Autodesk Fusion 360 part; units mm, degrees
note: some values were not read from the file. Set by a fixed rule: which face or edge a step refers to.
(part 3 of 4)
sketch "Sketch73" plane through (0, 0, 76.2) normal (0, 0, 1) x (1, 0, 0)
  line L0 (-231.5, 328) -> (-231.5, 317.5)
  line L1 (-231.5, 317.5) -> (-83.5, 317.5)
  line L2 (-83.5, 317.5) -> (-83.5, 328)
  line L3 (-83.5, 328) -> (-231.5, 328)
  circle A0 through (-77.5, 207.5, -7.5) (-80.5, 209.2321, -7.5) (-80.5, 205.7679, -7.5)
  circle A1 through (-77.5, 207.5, -7.5) (-80.5, 209.2321, -7.5) (-80.5, 205.7679, -7.5)
  circle A2 through (-77.5, 323.5, -7.5) (-80.5, 325.2321, -7.5) (-80.5, 321.7679, -7.5)
  circle A3 through (-77.5, 323.5, -7.5) (-80.5, 325.2321, -7.5) (-80.5, 321.7679, -7.5)
  circle A4 through (-233.5, 207.5, -25) (-236.5, 209.2321, -25) (-236.5, 205.7679, -25)
  circle A5 through (-233.5, 207.5, -25) (-236.5, 209.2321, -25) (-236.5, 205.7679, -25)
  circle A6 through (-233.5, 323.5, -25) (-236.5, 325.2321, -25) (-236.5, 321.7679, -25)
  circle A7 through (-233.5, 323.5, -25) (-236.5, 325.2321, -25) (-236.5, 321.7679, -25)
  circle A8 through (-77.5, 323.5, -25) (-80.5, 325.2321, -25) (-80.5, 321.7679, -25)
  circle A9 through (-77.5, 323.5, -25) (-80.5, 325.2321, -25) (-80.5, 321.7679, -25)
  circle A10 through (-77.5, 207.5, -25) (-80.5, 209.2321, -25) (-80.5, 205.7679, -25)
  circle A11 through (-77.5, 207.5, -25) (-80.5, 209.2321, -25) (-80.5, 205.7679, -25)
  point P0 (-235.5, 205.5)
sketch "Sketch74" plane through (0, 0, 76.2) normal (0, 0, 1) x (1, 0, 0)
  line L0 (-231.5, 213.5) -> (-231.5, 203)
  line L1 (-231.5, 203) -> (-83.5, 203)
  line L2 (-83.5, 203) -> (-83.5, 213.5)
  line L3 (-83.5, 213.5) -> (-231.5, 213.5)
  line L4 (-70, 213.5) -> (-140, 213.5)
  line L5 (-140, 213.5) -> (-140, 209.5)
  line L6 (-140, 209.5) -> (-70, 209.5)
  line L7 (-70, 209.5) -> (-70, 213.5)
  line L8 (-140, 209.5) -> (-175, 209.5)
  line L9 (-175, 209.5) -> (-175, 213.5)
  line L10 (-175, 213.5) -> (-140, 213.5)
  line L11 (-140, 213.5) -> (-140, 209.5)
  point P0 (-70, 213.5)
  dimension "d493" = 70
  dimension "d494" = 4
  dimension "d495" = 35
  constraint horizontal L4
  constraint vertical L5
  constraint horizontal L6
  constraint vertical L7
  constraint coincident P0 L4.start
  constraint horizontal L8
  constraint vertical L9
  constraint horizontal L10
  constraint vertical L11
  measures "d493" distance of P0 L4.end
  measures "d494" distance of P0 L6.end
  measures "d495" distance of L5.end L8.end
extrude "Extrude189" cut sketch "Sketch74" against normal blind 7.5 contours L3 L5 L8 L9 L10 L11 bodies 1
extrude "Extrude190" cut 1 faces at (-249.7333, 234.8333, 69.7) along direction (0, 0, 1) blind 2 on bodies 1 bodies 1
sketch "Sketch75" plane through (0, 213.5, 0) normal (0, 1, 0) x (-1, 0, 0)
  line L0 (175, 76.2) -> (175, 68.7)
  line L1 (175, 68.7) -> (140, 68.7)
  line L2 (140, 68.7) -> (140, 76.2)
  line L3 (140, 76.2) -> (83.5, 76.2)
  line L4 (83.5, 76.2) -> (83.5, 68.7)
  line L5 (83.5, 68.7) -> (74.5, 68.7)
  line L6 (74.5, 68.7) -> (74.5, 76.2)
  line L7 (74.5, 76.2) -> (70, 76.2)
  line L8 (70, 76.2) -> (70, 51.2)
  line L9 (245, 51.2) -> (245, 59.7)
  line L10 (245, 59.7) -> (267.2, 59.7)
  line L11 (267.2, 59.7) -> (257.6, 71.7)
  line L12 (257.6, 71.7) -> (245, 71.7)
  line L13 (245, 71.7) -> (245, 76.2)
  line L14 (245, 76.2) -> (240.5, 76.2)
  line L15 (240.5, 76.2) -> (240.5, 68.7)
  line L16 (240.5, 68.7) -> (231.5, 68.7)
  line L17 (231.5, 68.7) -> (231.5, 76.2)
  line L18 (231.5, 76.2) -> (175, 76.2)
extrude "Extrude191" cut 1 faces at (-252.4, 256.1667, 59.7) along direction (0, 0, -1) blind 2 on bodies 1 bodies 1
sketch "Sketch76" plane through (-192.0488, 0, 153.639) normal (-0.780869, 0, 0.624695) x (0.624695, 0, 0.780869)
  line L0 (-99.1703, 328) -> (-124.7828, 328)
  line L1 (-124.7828, 0) -> (-99.1703, 0)
  line L2 (-99.1703, 0) -> (-99.1703, 5)
  line L3 (-99.1703, 5) -> (-99.1703, 203)
  line L4 (-99.1703, 203) -> (-99.1703, 328)
  line L5 (-120.3006, 277.5) -> (-104.9332, 277.5)
  line L6 (-104.9332, 277.5) -> (-104.9332, 213.5)
  line L7 (-104.9332, 213.5) -> (-120.3006, 213.5)
sketch "Sketch77" plane through (0, 0, 57.7) normal (0, 0, 1) x (1, 0, 0)
  line L0 (-267.2, 277.5) -> (-267.2, 213.5)
  line L1 (-267.2, 213.5) -> (-245, 213.5)
  line L2 (-245, 213.5) -> (-245, 277.5)
  line L3 (-245, 277.5) -> (-267.2, 277.5)
  line L4 (-245, 213.5) -> (-254, 213.5)
  line L5 (-254, 213.5) -> (-254, 277.5)
  line L6 (-254, 277.5) -> (-245, 277.5)
  line L7 (-245, 277.5) -> (-245, 213.5)
  line L8 (-257.6, 213.5, 14) -> (-307.6, 213.5, 14)
  line L9 (-307.6, 213.5, 14) -> (-307.6, 277.5, 14)
  line L10 (-307.6, 277.5, 14) -> (-257.6, 277.5, 14)
  line L11 (-257.6, 277.5, 14) -> (-257.6, 213.5, 14)
  line L12 (-257.6, 277.5, 14) -> (-307.6, 277.5, 14)
  line L13 (-307.6, 277.5, 14) -> (-307.6, 287.5, 14)
  line L14 (-307.6, 287.5, 14) -> (-257.6, 287.5, 14)
  line L15 (-257.6, 287.5, 14) -> (-257.6, 277.5, 14)
  line L16 (-307.6, 213.5, 14) -> (-257.6, 213.5, 14)
  line L17 (-257.6, 213.5, 14) -> (-257.6, 203.5, 14)
  line L18 (-257.6, 203.5, 14) -> (-307.6, 203.5, 14)
  line L19 (-307.6, 203.5, 14) -> (-307.6, 213.5, 14)
  line L20 (-307.6, 287.5, 14) -> (-317.6, 287.5, 14)
  line L21 (-317.6, 287.5, 14) -> (-317.6, 203.5, 14)
  line L22 (-317.6, 203.5, 14) -> (-307.6, 203.5, 14)
  line L23 (-307.6, 203.5, 14) -> (-307.6, 287.5, 14)
  point P0 (-257.6, 213.5)
  dimension "d502" = 9
  dimension "d503" = 50
  dimension "d504" = 10
  dimension "d505" = 10
  dimension "d506" = 10
  constraint horizontal L4
  constraint vertical L5
  constraint horizontal L6
  constraint vertical L7
  constraint coincident L1.end L2.start
  measures "d502" distance of L1.end L4.end
extrude "Extrude192" add sketch "Sketch77" against normal blind 72 separate body contours L9 L13 L19 L20 L21 L22 L23 in plane through (0, 0, 71.7) normal (0, 0, 1) makes body 4
extrude "Extrude193" cut 1 faces at (-267.2, 234.8333, 59.0333) along direction (-1, 0, 0) blind 7 on bodies 1 bodies 1
sketch "Sketch78" plane through (0, 0, 71.7) normal (0, 0, 1) x (1, 0, 0)
  line L0 (-307.6, 203.5) -> (-307.6, 287.5)
  line L1 (-307.6, 287.5) -> (-317.6, 287.5)
  line L2 (-317.6, 287.5) -> (-317.6, 203.5)
  line L3 (-317.6, 203.5) -> (-307.6, 203.5)
  line L4 (-257.6, 277.5) -> (-307.6, 277.5)
  line L5 (-257.6, 213.5) -> (-307.6, 213.5)
  line L6 (-257.6, 213.5, 0) -> (-268.8, 213.5, -14)
  line L7 (-307.6, 277.5) -> (-268.8, 277.5)
  line L8 (-268.8, 277.5, 0) -> (-268.8, 277.5, -14)
  line L9 (-268.8, 277.5, -14) -> (-307.6, 277.5, -14)
  line L10 (-307.6, 277.5, -14) -> (-307.6, 277.5, 0)
  line L11 (-307.6, 213.5) -> (-268.8, 213.5)
  line L12 (-268.8, 213.5, 0) -> (-268.8, 213.5, -14)
  line L13 (-268.8, 213.5, -14) -> (-307.6, 213.5, -14)
  line L14 (-307.6, 213.5, -14) -> (-307.6, 213.5, 0)
  point P0 (-257.6, 277.5)
  point P1 (-257.6, 213.5)
  point P2 (-257.6, 213.5)
  point P3 (-268.8, 213.5)
  point P4 (-268.8, 277.5)
  constraint coincident P0 L4.start
  constraint coincident L0 L4.end
  constraint perpendicular L0 L4
  constraint coincident P2 P1
  constraint coincident L0 L5.end
  constraint perpendicular L0 L5
  constraint coincident P3 L11.end
  constraint horizontal L7
  constraint coincident P4 L7.end
  constraint horizontal L11
extrude "Extrude194" add sketch "Sketch78" against normal blind 10 contours L5 L6 L12 | L5 L11 L12 L13 L14 in plane through (0, 213.5, 71.7) normal (0, 1, 0) bodies 4 1
sketch "Sketch79" plane through (0, 287.5, 0) normal (0, 1, 0) x (-1, 0, 0)
  line L0 (317.6, 71.7) -> (307.6, 71.7)
  line L1 (307.6, 71.7) -> (307.6, -0.3)
  line L2 (307.6, -0.3) -> (317.6, -0.3)
  line L3 (317.6, -0.3) -> (317.6, 71.7)
  line L4 (307.6, 71.7, -74) -> (307.6, 71.7, 0)
  line L5 (257.6, 71.7, -10) -> (307.6, 71.7, -10)
  line L6 (268.8, 57.7, -10) -> (257.6, 71.7, -10)
  line L7 (268.8, 57.7, -10) -> (307.6, 57.7, -10)
  line L8 (307.6, 57.7, -10) -> (307.6, 71.7, -10)
  line L9 (307.6, 71.7, -10) -> (268.8, 71.7, -10)
  line L10 (268.8, 71.7, -10) -> (268.8, 57.7, -10)
  point P0 (257.6, 71.7)
  point P1 (268.8, 57.7)
  point P2 (257.6, 71.7)
  constraint coincident P2 P0
extrude "Extrude195" add sketch "Sketch79" along normal blind 10 separate body contours L5 L6 L10 | L5 L7 L8 L9 L10 in plane through (0, 277.5, 0) normal (0, 1, 0) makes body 5
sketch "Sketch80" plane through (-317.6, 0, 0) normal (-1, 0, 0) x (0, 0, 1)
sketch "Sketch81" plane through (0, 203.5, 0) normal (0, -1, 0) x (1, 0, 0)
  line L0 (-257.6, 71.7) -> (-317.6, 71.7)
  line L1 (-317.6, 71.7) -> (-317.6, -0.3)
  line L2 (-317.6, -0.3) -> (-307.6, -0.3)
  line L3 (-307.6, -0.3) -> (-307.6, 57.7)
  line L4 (-307.6, 57.7) -> (-268.8, 57.7)
  line L5 (-268.8, 57.7) -> (-257.6, 71.7)
  line L6 (-268.8, 57.7) -> (-307.6, 57.7)
  line L7 (-270, 56.2, -124.5) -> (-270, 56.2, 203.5)
  line L8 (-268.8, 57.7) -> (-270, 56.2)
  line L9 (-307.6, 57.7) -> (-270, 57.7)
  line L10 (-270, 57.7) -> (-270, 56.2)
  line L11 (-270, 56.2) -> (-307.6, 56.2)
  line L12 (-307.6, 56.2) -> (-307.6, 57.7)
  line L13 (-279, 0, -124.5) -> (-279, 10, -124.5)
  line L14 (-279, 10, -124.5) -> (-279, 10, -84)
  line L15 (-279, 10, -84) -> (-279, 0, -84)
  line L16 (-279, 0, -84) -> (-279, 0, -124.5)
  line L17 (-279, 0, -84) -> (-317.6, 0, -84)
  line L18 (-317.6, 0, -84) -> (-317.6, 10, -84)
  line L19 (-317.6, 10, -84) -> (-279, 10, -84)
  line L20 (-279, 10, -84) -> (-279, 0, -84)
  line L21 (-307.6, 10, -84) -> (-307.6, 0, -84)
  point P0 (-279, 0)
  dimension "d515" = 10
  dimension "d516" = 40.5
  dimension "d517" = 10
  constraint coincident L4.end L5.start
  constraint coincident L3.end L4.start
  constraint parallel L5 L8
  constraint horizontal L9
  constraint vertical L10
  constraint horizontal L11
  constraint vertical L12
extrude "Extrude196" add sketch "Sketch81" along normal blind 84.001 separate body contours L15 L17 L19 L20 L21 in plane through (0, 287.5, 0) normal (0, -1, 0) makes body 6
sketch "Sketch82" plane through (0, 0, 76.2) normal (0, 0, 1) x (1, 0, 0)
  line L0 (-240.5, 203) -> (-240.5, 213.5)
  line L1 (-240.5, 213.5) -> (-245, 213.5)
  line L2 (-245, 213.5) -> (-245, 317.5)
  line L3 (-245, 317.5) -> (-240.5, 317.5)
  line L4 (-240.5, 317.5) -> (-240.5, 328)
  line L5 (-240.5, 328) -> (-254, 328)
  line L6 (-254, 328) -> (-254, 203)
  line L7 (-254, 203) -> (-240.5, 203)
  line L8 (-245, 277.5, -18.5) -> (-307.6, 277.5, -18.5)
  line L9 (-307.6, 277.5, -18.5) -> (-307.6, 213.5, -18.5)
  line L10 (-307.6, 213.5, -18.5) -> (-245, 213.5, -18.5)
  line L11 (-245, 213.5, -18.5) -> (-245, 277.5, -18.5)
  point P0 (-245, 277.5)
  point P1 (-307.6, 213.5)
extrude "Extrude197" cut sketch "Sketch82" against normal blind 50 contours L8 L9 L10 L11 in plane through (0, 0, 57.7) normal (0, 0, 1) bodies 4 6
sketch "Sketch83" plane through (0, 213.5, 0) normal (0, 1, 0) x (-1, 0, 0)
  line L0 (175, 76.2) -> (175, 68.7)
  line L1 (175, 68.7) -> (140, 68.7)
  line L2 (140, 68.7) -> (140, 76.2)
  line L3 (140, 76.2) -> (83.5, 76.2)
  line L4 (83.5, 76.2) -> (83.5, 68.7)
  line L5 (83.5, 68.7) -> (74.5, 68.7)
  line L6 (74.5, 68.7) -> (74.5, 76.2)
  line L7 (74.5, 76.2) -> (70, 76.2)
  line L8 (70, 76.2) -> (70, 51.2)
  line L9 (70, 51.2) -> (254, 51.2)
  line L10 (254, 51.2) -> (254, 20)
  line L11 (254, 20) -> (245, 20)
  line L12 (245, 20) -> (245, 15.5)
  line L13 (245, 15.5) -> (247, 15.5)
  line L14 (247, 15.5) -> (247, 10)
  line L15 (247, 10) -> (254, 10)
  line L16 (254, 10) -> (254, 7.7)
  line L17 (254, 7.7) -> (279, 7.7)
  line L18 (279, 7.7) -> (279, 36.1286)
  line L19 (279, 36.1286) -> (270, 45.1607)
  line L20 (270, 45.1607) -> (270, 56.2)
  line L21 (270, 56.2) -> (268.8, 57.7)
  line L22 (268.8, 57.7) -> (307.6, 57.7)
  line L23 (307.6, 57.7) -> (307.6, 71.7)
  line L24 (307.6, 71.7) -> (257.6, 71.7)
  line L25 (257.6, 71.7) -> (245, 71.7)
  line L26 (245, 71.7) -> (245, 76.2)
  line L27 (245, 76.2) -> (240.5, 76.2)
  line L28 (240.5, 76.2) -> (240.5, 68.7)
  line L29 (240.5, 68.7) -> (231.5, 68.7)
  line L30 (231.5, 68.7) -> (231.5, 76.2)
  line L31 (231.5, 76.2) -> (175, 76.2)
  line L32 (279, 10) -> (307.6, 10)
  line L33 (307.6, 10) -> (307.6, 57.7)
  line L34 (307.6, 57.7) -> (279, 57.7)
  line L35 (279, 57.7) -> (279, 10)
  point P0 (279, 10)
  constraint horizontal L32
  constraint vertical L33
  constraint horizontal L34
  constraint vertical L35
  constraint coincident L22.end L23.start
  constraint coincident P0 L32.start
extrude "Extrude198" add sketch "Sketch83" against normal blind 10 contours L18 L22 L32 L33 L34 L35 bodies 6 5 4
sketch "Sketch84" plane through (0, 213.5, 0) normal (0, 1, 0) x (-1, 0, 0)
  line L0 (307.6, 7.7) -> (307.6, 71.7)
  line L1 (307.6, 71.7) -> (257.6, 71.7)
  line L2 (257.6, 71.7) -> (245, 71.7)
  line L3 (245, 71.7) -> (245, 76.2)
  line L4 (245, 76.2) -> (240.5, 76.2)
  line L5 (240.5, 76.2) -> (240.5, 68.7)
  line L6 (240.5, 68.7) -> (231.5, 68.7)
  line L7 (231.5, 68.7) -> (231.5, 76.2)
  line L8 (231.5, 76.2) -> (175, 76.2)
  line L9 (175, 76.2) -> (175, 68.7)
  line L10 (175, 68.7) -> (140, 68.7)
  line L11 (140, 68.7) -> (140, 76.2)
  line L12 (140, 76.2) -> (83.5, 76.2)
  line L13 (83.5, 76.2) -> (83.5, 68.7)
  line L14 (83.5, 68.7) -> (74.5, 68.7)
  line L15 (74.5, 68.7) -> (74.5, 76.2)
  line L16 (74.5, 76.2) -> (70, 76.2)
  line L17 (70, 76.2) -> (70, 51.2)
  line L18 (70, 51.2) -> (254, 51.2)
  line L19 (254, 51.2) -> (254, 20)
  line L20 (254, 20) -> (245, 20)
  line L21 (245, 20) -> (245, 15.5)
  line L22 (245, 15.5) -> (247, 15.5)
  line L23 (247, 15.5) -> (247, 10)
  line L24 (247, 10) -> (254, 10)
  line L25 (254, 10) -> (254, 7.7)
  line L26 (254, 7.7) -> (307.6, 7.7)
  line L27 (279, 36.1286) -> (270, 45.1607)
  line L28 (270, 56.2) -> (268.8, 57.7)
  line L29 (268.8, 57.7) -> (279, 57.7)
extrude "Extrude199" cut 1 faces at (-275.6, 206.8333, 57.7) along direction (0, 0, -1) blind 2 on bodies 6 bodies 6
extrude "Extrude200" add 1 faces at (-275.6, 206.8333, 57.7) along direction (0, 0, -1) blind 2 on bodies 6 bodies 6
sketch "Sketch85" plane through (0, 203.5, 0) normal (0, -1, 0) x (1, 0, 0)
  line L0 (-257.6, 71.7) -> (-317.6, 71.7)
  line L1 (-317.6, 71.7) -> (-317.6, -0.3)
  line L2 (-317.6, -0.3) -> (-307.6, -0.3)
  line L3 (-307.6, -0.3) -> (-307.6, 0)
  line L4 (-307.6, 0) -> (-307.6, 10)
  line L5 (-307.6, 10) -> (-279, 10)
  line L6 (-279, 10) -> (-279, 36.1286)
  line L7 (-279, 36.1286) -> (-279, 55.7)
  line L8 (-279, 55.7) -> (-270, 55.7)
  line L9 (-270, 55.7) -> (-270, 56.2)
  line L10 (-270, 56.2) -> (-257.6, 71.7)
  line L11 (-270, 55.7) -> (-279, 55.7)
  line L12 (-279, 55.7) -> (-279, 36.1286)
  line L13 (-270, 45.1607, 203.5) -> (-270, 45.1607, -10)
  line L14 (-279, 36.1286) -> (-270, 45.1607)
  line L15 (-270, 55.7) -> (-270, 45.1607)
  constraint coincident L8.end L9.start
  constraint coincident L7.end L8.start
  constraint coincident L6.end L7.start
extrude "Extrude201" add sketch "Sketch85" against normal blind 10 separate body contours L7 L8 L11 L12 L14 L15 makes body 7
extrude "Extrude202" cut 3 faces at (-301.4, 203.5, 39.2762) (-288.5333, 203.4993, 10) (-307.6, 203.4997, 6.6667) along direction (0, 1, 0) blind 3 on bodies 6 bodies 6
extrude "Extrude203" cut 1 faces at (-298.0667, 203.499, 6.6667) along direction (0, 1, 0) blind 3 on bodies 6 bodies 6
extrude "Extrude204" cut 1 faces at (-276, 203.5, 45.6631) along direction (0, 1, 0) blind 3 on bodies 7 bodies 7
extrude "Extrude205" cut 1 faces at (-317.6, 260.5, 23.7) along direction (1, 0, 0) blind 3 on bodies 6 bodies 6
sketch "Sketch86" plane through (0, 213.5, 0) normal (0, 1, 0) x (-1, 0, 0)
  line L0 (279, 10, 74) -> (307.6, 10, 74)
  line L1 (307.6, 10, 74) -> (307.6, 57.7, 74)
  line L2 (307.6, 57.7, 74) -> (279, 57.7, 74)
  line L3 (279, 57.7, 74) -> (279, 10, 74)
  line L4 (268.8, 57.7, 74) -> (279, 57.7, 74)
  point P0 (279, 10)
  point P1 (307.6, 57.7)
  point P2 (268.8, 57.7)
extrude "Extrude206" add sketch "Sketch86" against normal blind 10 contours L0 L1 L2 L3 in plane through (0, 287.5, 0) normal (0, 1, 0) bodies 5 7 6
sketch "Sketch87" plane through (0, 287.5, 0) normal (0, 1, 0) x (-1, 0, 0)
  line L0 (268.8, 57.7) -> (279, 57.7)
  line L1 (279, 57.7) -> (279, 36.1286)
  line L2 (279, 36.1286) -> (279, 0)
  line L3 (279, 0) -> (307.6, 0)
  line L4 (307.6, 0) -> (307.6, -0.3)
  line L5 (307.6, -0.3) -> (314.6, -0.3)
  line L6 (314.6, -0.3) -> (314.6, 71.7)
  line L7 (314.6, 71.7) -> (257.6, 71.7)
  line L8 (257.6, 71.7) -> (268.8, 57.7)
  line L9 (268.8, 57.7, -10) -> (268.8, 57.7, 0)
  line L10 (268.8, 57.7) -> (270, 56.2)
  line L11 (270, 56.2) -> (270, 57.7)
  point P0 (270, 45.1607)
  point P1 (270, 45.1607)
  point P2 (270, 56.2)
  point P3 (270, 56.2)
  point P4 (268.8, 57.7)
  constraint coincident P4 L0.start
  constraint parallel L8 L10
  constraint coincident L0 L11.end
  constraint perpendicular L0 L11
extrude "Extrude207" add sketch "Sketch87" against normal blind 10 separate body contours L0 L10 L11 makes body 8
sketch "Sketch88" plane through (0, 287.5, 0) normal (0, 1, 0) x (-1, 0, 0)
  line L0 (279, 36.1286) -> (279, 0)
  line L1 (279, 0) -> (307.6, 0)
  line L2 (307.6, 0) -> (307.6, -0.3)
  line L3 (307.6, -0.3) -> (314.6, -0.3)
  line L4 (314.6, -0.3) -> (314.6, 71.7)
extrude "Extrude208" add 1 faces at (-270, 284.1667, 56.7) along direction (-1, 0, 0) blind 9 on bodies 8 bodies 8 7 5
extrude "Extrude209" add 1 faces at (-270, 297.6667, 48.8405) along direction (-1, 0, 0) blind 9 on bodies 8 bodies 8
sketch "Sketch89" plane through (0, 328, 0) normal (0, 1, 0) x (-1, 0, 0)
  line L0 (231.5, 68.7) -> (231.5, 76.2)
  line L1 (231.5, 76.2) -> (83.5, 76.2)
  line L2 (83.5, 76.2) -> (83.5, 68.7)
  line L3 (83.5, 68.7) -> (74.5, 68.7)
  line L4 (74.5, 68.7) -> (74.5, 76.2)
  line L5 (74.5, 76.2) -> (61, 76.2)
  line L6 (61, 76.2) -> (45, 56.1607)
  line L7 (45, 56.1607) -> (53.7273, 56.1821)
  line L8 (53.7273, 56.1821) -> (51, 56.1607)
  line L9 (51, 56.1607) -> (45, 56.1607)
  line L10 (45, 56.1607) -> (45, 45.1607)
  line L11 (45, 45.1607) -> (36, 36.1286)
  line L12 (36, 36.1286) -> (36, 0)
  line L13 (36, 0) -> (56, 0)
  line L14 (56, 0) -> (56, -71)
  line L15 (56, -71) -> (61, -71)
  line L16 (61, -71) -> (61, 51.2)
  line L17 (61, 51.2) -> (254, 51.2)
  line L18 (254, 51.2) -> (254, -71)
  line L19 (254, -71) -> (259, -71)
  line L20 (259, -71) -> (259, 0)
  line L21 (259, 0) -> (279, 0)
  line L22 (279, 0) -> (279, 36.1286)
  line L23 (279, 36.1286) -> (270, 45.1607)
  line L24 (270, 45.1607) -> (279, 45.1607)
  line L25 (279, 45.1607) -> (279, 56.2)
  line L26 (279, 56.2) -> (270, 56.2)
  line L27 (270, 56.2) -> (254, 76.2)
  line L28 (254, 76.2) -> (240.5, 76.2)
  line L29 (240.5, 76.2) -> (240.5, 68.7)
  line L30 (240.5, 68.7) -> (231.5, 68.7)
  line L31 (270, 56.2) -> (279, 56.2)
  line L32 (279, 56.2) -> (279, 36.1286)
  line L33 (279, 36.1286) -> (270, 36.1286)
  line L34 (270, 36.1286) -> (270, 56.2)
  line L35 (270, 45.1607) -> (279, 45.1607)
  line L36 (270, 45.1607) -> (279, 36.1286)
  constraint horizontal L31
  constraint vertical L32
  constraint horizontal L33
  constraint vertical L34
  constraint coincident L22.end L23.start
  constraint coincident L26.end L27.start
  constraint coincident L23.end L24.start
  constraint coincident L24.end L25.start
extrude "Extrude210" add sketch "Sketch89" against normal blind 50.5 separate body contours L23 L24 L32 L35 L36 makes body 9
sketch "Sketch90" plane through (0, 328, 0) normal (0, 1, 0) x (-1, 0, 0)
  line L0 (231.5, 68.7) -> (231.5, 76.2)
  line L1 (231.5, 76.2) -> (83.5, 76.2)
  line L2 (83.5, 76.2) -> (83.5, 68.7)
  line L3 (83.5, 68.7) -> (74.5, 68.7)
  line L4 (74.5, 68.7) -> (74.5, 76.2)
  line L5 (74.5, 76.2) -> (61, 76.2)
  line L6 (61, 76.2) -> (45, 56.1607)
  line L7 (45, 56.1607) -> (53.7273, 56.1821)
  line L8 (53.7273, 56.1821) -> (51, 56.1607)
  line L9 (51, 56.1607) -> (45, 56.1607)
  line L10 (45, 56.1607) -> (45, 45.1607)
  line L11 (45, 45.1607) -> (36, 36.1286)
  line L12 (36, 36.1286) -> (36, 0)
  line L13 (36, 0) -> (56, 0)
  line L14 (56, 0) -> (56, -71)
  line L15 (56, -71) -> (61, -71)
  line L16 (61, -71) -> (61, 51.2)
  line L17 (61, 51.2) -> (254, 51.2)
  line L18 (254, 51.2) -> (254, -71)
  line L19 (254, -71) -> (259, -71)
  line L20 (259, -71) -> (259, 0)
  line L21 (259, 0) -> (279, 0)
  line L22 (279, 0) -> (279, 36.1286)
  line L23 (279, 36.1286) -> (270, 45.1607)
  line L24 (270, 45.1607) -> (279, 45.1607)
  line L25 (279, 45.1607) -> (279, 56.2)
  line L26 (279, 56.2) -> (270, 56.2)
  line L27 (270, 56.2) -> (254, 76.2)
  line L28 (254, 76.2) -> (240.5, 76.2)
  line L29 (240.5, 76.2) -> (240.5, 68.7)
  line L30 (240.5, 68.7) -> (231.5, 68.7)
  line L31 (279, 56.2) -> (259, 56.2)
  line L32 (259, 56.2) -> (259, 0)
  line L33 (259, 0) -> (279, 0)
  line L34 (279, 0) -> (279, 56.2)
  constraint horizontal L31
  constraint vertical L32
  constraint horizontal L33
  constraint vertical L34
  constraint coincident L20.end L21.start
  constraint coincident L25.end L26.start
extrude "Extrude211" cut sketch "Sketch90" against normal blind 40 contours L21 L22 L23 L24 L25 L26 L31 L32 L33 L34 | L23 L24 L34 bodies 8 9
extrude "Extrude212" cut 1 faces at (-272.3333, 288, 12.0429) along direction (0, -1, 0) blind 10 on bodies 8 bodies 8
extrude "Extrude213" cut 1 faces at (-276, 288, 42.15) along direction (0, -1, 0) blind 10 on bodies 9 bodies 9
extrude "Extrude214" cut 1 faces at (-272.3333, 278, 12.0429) along direction (0, -1, 0) blind 3 on bodies 8 bodies 8
extrude "Extrude215" cut 1 faces at (-276, 277.5, 42.15) along direction (0, 1, 0) blind 2 on bodies 9 bodies 9
extrude "Extrude216" cut 1 faces at (-262.6667, 297.6667, 56.2) along direction (0, 0, 1) blind 20 on bodies 8 bodies 8
extrude "Extrude217" add 1 faces at (-265.6667, 275, 5.1333) along direction (0, 1, 0) blind 12.5 on bodies 8 bodies 8 9
sketch "Sketch91" plane through (0, 287.5, 0) normal (0, 1, 0) x (-1, 0, 0)
  line L0 (259, 69.95) -> (259, 71.7)
  line L1 (259, 69.95) -> (257.6, 71.7)
  line L2 (257.6, 71.7) -> (259, 71.7)
  point P0 (259, 69.95)
  point P1 (259, 71.7)
  point P2 (257.6, 71.7)
  constraint coincident P0 L0.start
  constraint coincident P1 L0.end
  constraint coincident P2 L1.end
extrude "Extrude218" cut sketch "Sketch91" against normal blind 11.8 bodies 8
extrude "Extrude219" add 1 faces at (-279, 284.1667, 50.3667) along direction (1, 0, 0) blind 20 on bodies 8 bodies 8
extrude "Extrude220" cut 1 faces at (-293.7333, 284.1667, 71.7) along direction (0, 0, -1) blind 2 on bodies 8 bodies 8
sketch "Sketch92" plane through (0, 0, 69.7) normal (0, 0, 1) x (1, 0, 0)
  line L0 (-259, 287.5) -> (-314.6, 287.5)
  line L1 (-314.6, 287.5) -> (-314.6, 206.5)
  line L2 (-314.6, 206.5) -> (-259.2, 206.5)
  line L3 (-259.2, 206.5) -> (-257.6, 206.5)
  line L4 (-257.6, 206.5) -> (-257.6, 213.5)
  line L5 (-257.6, 213.5) -> (-307.6, 213.5)
  line L6 (-307.6, 213.5) -> (-307.6, 277.5)
  line L7 (-307.6, 277.5) -> (-259, 277.5)
  line L8 (-259, 277.5) -> (-259, 287.5)
  line L9 (-257.6, 213.5) -> (-307.6, 213.5)
  line L10 (-307.6, 213.5) -> (-307.6, 277.5)
  line L11 (-307.6, 277.5) -> (-257.6, 277.5)
  line L12 (-257.6, 277.5) -> (-257.6, 213.5)
  constraint horizontal L9
  constraint vertical L10
  constraint horizontal L11
  constraint vertical L12
  constraint coincident L6.end L7.start
  constraint coincident L4.end L5.start
extrude "Extrude221" add sketch "Sketch92" along normal blind 5 separate body contours L5 L6 L7 L9 L10 L11 L12 makes body 10
extrude "Extrude222" cut 1 faces at (-274.7333, 234.8333, 74.7) along direction (0, 0, -1) blind 3 on bodies 10 bodies 10
extrude "Extrude223" add 1 faces at (-293.7333, 284.1667, 69.7) along direction (0, 0, 1) blind 2 on bodies 8 bodies 8 10
extrude "Extrude224" add 1 faces at (-258.5333, 277.5, 71.1167) along direction (0, 1, 0) blind 10 on bodies 8 bodies 8
extrude "Extrude225" cut 1 faces at (-281.8667, 260.4997, 0) along direction (0, 0, 1) blind 3 on bodies 8 bodies 8
extrude "Extrude226" cut 1 faces at (-312.2667, 260.5, -0.3) along direction (0, 0, 1) blind 3.3 on bodies 8 bodies 8
fillet "Fillet1" radius 8 1 edges at (-314.6, 247, 71.7) on bodies 8
fillet "Fillet2" radius 8 1 edges at (-314.6, 247, 3) on bodies 8
fillet "Fillet3" radius 8 5 edges at (-282.8, 287.5, 3) (-312.2569, 287.5, 5.3431) (-314.6, 287.5, 37.35) (-312.2569, 287.5, 69.3569) (-282.1, 287.5, 71.7) on bodies 8
fillet "Fillet4" radius 4 4 edges at (-282.1, 206.5, 71.7) (-312.2569, 206.5, 69.3569) (-314.6, 206.5, 37.35) (-312.6, 206.5, 5.7085) on bodies 8
sketch "Sketch93" plane through (0, 0, 51.2) normal (0, 0, -1) x (-1, 0, 0)
  line L0 (254, 213.5) -> (70, 213.5)
  line L1 (70, 213.5) -> (70, 317.5)
  line L2 (70, 317.5) -> (245, 317.5)
  line L3 (245, 317.5) -> (245, 277.5)
  line L4 (245, 277.5) -> (254, 277.5)
  line L5 (254, 277.5) -> (254, 328)
  line L6 (254, 328) -> (61, 328)
  line L7 (61, 328) -> (61, 155)
  line L8 (61, 155) -> (66, 155)
  line L9 (66, 155) -> (66, 5)
  line L10 (66, 5) -> (89, 5)
  line L11 (89, 5) -> (89, 155)
  line L12 (89, 155) -> (96, 155)
  line L13 (96, 155) -> (96, 64.5)
  line L14 (96, 64.5) -> (219, 64.5)
  line L15 (219, 64.5) -> (219, 155)
  line L16 (219, 155) -> (226.5, 155)
  line L17 (226.5, 155) -> (226.5, 135)
  line L18 (226.5, 135) -> (223, 135)
  line L19 (223, 135) -> (223, 60.5)
  line L20 (223, 60.5) -> (218, 60.5)
  line L21 (218, 60.5) -> (218, 5)
  line L22 (218, 5) -> (250.5, 5)
  line L23 (250.5, 5) -> (250.5, 155)
  line L24 (250.5, 155) -> (254, 155)
  line L25 (254, 155) -> (254, 213.5)
  circle A0 centre (235.5, 323.5) radius 2
  circle A1 centre (79.5, 323.5) radius 2
  circle A2 centre (229, 25) radius 6.15
  circle A3 centre (235.5, 207.5) radius 2
  circle A4 centre (79.5, 207.5) radius 2
  line L26 (254, 317.5) -> (61, 317.5)
  line L27 (61, 317.5) -> (61, 328)
  line L28 (61, 328) -> (254, 328)
  line L29 (254, 328) -> (254, 317.5)
  constraint horizontal L26
  constraint vertical L27
  constraint horizontal L28
  constraint vertical L29
  constraint coincident L6.end L7.start
  constraint coincident L5 L26.start
extrude "Extrude227" cut sketch "Sketch93" against normal blind 5 contours L2 L5 L6 L7 L26 L27 L28 L29 bodies 8
sketch "Sketch94" plane through (0, 0, 51.2) normal (0, 0, -1) x (-1, 0, 0)
  circle A0 centre (79.5, 207.5) radius 2
  circle A1 centre (235.5, 207.5) radius 2
  circle A2 centre (229, 25) radius 6.15
  line L0 (70, 317.5) -> (61, 317.5)
  line L1 (61, 317.5) -> (61, 155)
  line L2 (61, 155) -> (66, 155)
  line L3 (66, 155) -> (66, 5)
  line L4 (66, 5) -> (89, 5)
  line L5 (89, 5) -> (89, 155)
  line L6 (89, 155) -> (96, 155)
  line L7 (96, 155) -> (96, 64.5)
  line L8 (96, 64.5) -> (219, 64.5)
  line L9 (219, 64.5) -> (219, 155)
  line L10 (219, 155) -> (226.5, 155)
  line L11 (226.5, 155) -> (226.5, 135)
  line L12 (226.5, 135) -> (223, 135)
  line L13 (223, 135) -> (223, 60.5)
  line L14 (223, 60.5) -> (218, 60.5)
  line L15 (218, 60.5) -> (218, 5)
  line L16 (218, 5) -> (250.5, 5)
  line L17 (250.5, 5) -> (250.5, 155)
  line L18 (250.5, 155) -> (254, 155)
  line L19 (254, 155) -> (254, 213.5)
  line L20 (254, 213.5) -> (70, 213.5)
  line L21 (70, 213.5) -> (70, 317.5)
  line L22 (254, 213.5) -> (61, 213.5)
  line L23 (61, 213.5) -> (61, 201.5)
  line L24 (61, 201.5) -> (254, 201.5)
  line L25 (254, 201.5) -> (254, 213.5)
  dimension "d590" = 12
  constraint horizontal L22
  constraint vertical L23
  constraint horizontal L24
  constraint vertical L25
  constraint coincident L19.end L20.start
  measures "d590" distance of L19.end L24.end
extrude "Extrude228" add 1 faces at (-132.8333, 203, 60.3667) along direction (0, -1, 0) blind 10 on bodies 8 bodies 8
extrude "Extrude229" cut sketch "Sketch94" against normal blind 5 contours L1 L19 L20 L22 L23 L24 L25 bodies 8
extrude "Extrude230" cut 1 faces at (-64, 282.8333, 51.2) along direction (0, 0, 1) blind 5 on bodies 8 bodies 8
extrude "Extrude231" cut 1 faces at (-248, 304.1667, 51.2) along direction (0, 0, 1) blind 5 on bodies 8 bodies 8
extrude "Extrude232" add 1 faces at (-249.2, 234.8333, 71.7) along direction (0, 0, -1) blind 2 on bodies 8 bodies 8
sketch "Sketch95" plane through (0, 213.5, 0) normal (0, 1, 0) x (-1, 0, 0)
extrude "Extrude233" cut 1 faces at (-237.6667, 217, 15.1667) along direction (0, -1, 0) blind 3.5 on bodies 8 bodies 8
extrude "Extrude234" cut 1 faces at (-62.6667, 155, 30.4) along direction (0, -1, 0) blind 150 on bodies 8 bodies 8
sketch "Sketch96" plane through (0, 328, 0) normal (0, 1, 0) x (-1, 0, 0)
  line L0 (61, -71) -> (61, 56.2)
  line L1 (61, 56.2) -> (254, 56.2)
  line L2 (254, 56.2) -> (254, -71)
  line L3 (254, -71) -> (259, -71)
  line L4 (259, -71) -> (259, 69.95)
  line L5 (259, 69.95) -> (254, 76.2)
  line L6 (254, 76.2) -> (240.5, 76.2)
  line L7 (240.5, 76.2) -> (240.5, 68.7)
  line L8 (240.5, 68.7) -> (231.5, 68.7)
  line L9 (231.5, 68.7) -> (231.5, 76.2)
  line L10 (231.5, 76.2) -> (83.5, 76.2)
  line L11 (83.5, 76.2) -> (83.5, 68.7)
  line L12 (83.5, 68.7) -> (74.5, 68.7)
  line L13 (74.5, 68.7) -> (74.5, 76.2)
  line L14 (74.5, 76.2) -> (61, 76.2)
  line L15 (61, 76.2) -> (45, 56.1607)
  line L16 (45, 56.1607) -> (53.7273, 56.1821)
  line L17 (53.7273, 56.1821) -> (51, 56.1607)
  line L18 (51, 56.1607) -> (45, 56.1607)
  line L19 (45, 56.1607) -> (45, 45.1607)
  line L20 (45, 45.1607) -> (36, 36.1286)
  line L21 (36, 36.1286) -> (36, 0)
  line L22 (36, 0) -> (56, 0)
  line L23 (56, 0) -> (56, -71)
  line L24 (56, -71) -> (61, -71)
  line L25 (61, 56.2) -> (254, 56.2)
  line L26 (254, 56.2) -> (254, 61.2)
  line L27 (254, 61.2) -> (61, 61.2)
  line L28 (61, 61.2) -> (61, 56.2)
  dimension "d605" = 5
  constraint horizontal L25
  constraint vertical L26
  constraint horizontal L27
  constraint vertical L28
  constraint coincident L0.end L1.start
  measures "d605" distance of L0.end L27.end
extrude "Extrude235" add sketch "Sketch96" along normal blind 5 separate body contours L0 L2 L3 L4 L5 L6 L7 L8 L9 L10 L11 L12 L13 L14 L15 L19 L20 L21 L22 L23 L24 L26 L27 L28 makes body 11
sketch "Sketch97" plane through (0, 333, 0) normal (0, 1, 0) x (-1, 0, 0)
  line L0 (254, 61.2) -> (254, -71)
  line L1 (254, -71) -> (259, -71)
  line L2 (259, -71) -> (259, 69.95)
  line L3 (259, 69.95) -> (254, 76.2)
  line L4 (254, 76.2) -> (240.5, 76.2)
  line L5 (240.5, 76.2) -> (240.5, 68.7)
  line L6 (240.5, 68.7) -> (231.5, 68.7)
  line L7 (231.5, 68.7) -> (231.5, 76.2)
  line L8 (231.5, 76.2) -> (83.5, 76.2)
  line L9 (83.5, 76.2) -> (83.5, 68.7)
  line L10 (83.5, 68.7) -> (74.5, 68.7)
  line L11 (74.5, 68.7) -> (74.5, 76.2)
  line L12 (74.5, 76.2) -> (61, 76.2)
  line L13 (61, 76.2) -> (45, 56.1607)
  line L14 (45, 56.1607) -> (53.7273, 56.1821)
  line L15 (53.7273, 56.1821) -> (51, 56.1607)
  line L16 (51, 56.1607) -> (45, 56.1607)
  line L17 (45, 56.1607) -> (45, 45.1607)
  line L18 (45, 45.1607) -> (36, 36.1286)
  line L19 (36, 36.1286) -> (36, 0)
  line L20 (36, 0) -> (56, 0)
  line L21 (56, 0) -> (56, -71)
  line L22 (56, -71) -> (61, -71)
  line L23 (61, -71) -> (61, 61.2)
  line L24 (61, 61.2) -> (254, 61.2)
  line L25 (61, 61.2) -> (56, 61.2)
  line L26 (56, 61.2) -> (56, -71)
  line L27 (56, -71) -> (61, -71)
  line L28 (61, -71) -> (61, 61.2)
  constraint horizontal L25
  constraint vertical L26
  constraint horizontal L27
  constraint vertical L28
  constraint coincident L21.end L22.start
  constraint coincident L23.end L24.start
extrude "Extrude236" cut sketch "Sketch97" against normal blind 5 contours L21 L22 L23 L25 L26 L27 L28 bodies 11
sketch "Sketch98" plane through (0, 0, 76.2) normal (0, 0, 1) x (1, 0, 0)
  line L0 (-254, 333, -15) -> (-259, 333, -15)
  line L1 (-259, 333, -15) -> (-259, 333, -147.2)
  line L2 (-259, 333, -147.2) -> (-254, 333, -147.2)
  line L3 (-254, 333, -147.2) -> (-254, 333, -15)
  point P0 (-254, 333)
  point P1 (-259, 333)
extrude "Extrude237" cut sketch "Sketch98" against normal blind 5 contours L0 L1 L2 L3 in plane through (0, 333, 76.2) normal (0, 1, 0) bodies 11
sketch "Sketch99" plane through (-259, 0, 0) normal (-1, 0, 0) x (0, 0, 1)
  line L0 (11, 287.5) -> (63.7, 287.5)
  arc A0 (69.95, 284.4937) -> (63.7, 287.5) centre (63.7, 279.5) ccw
  line L1 (69.95, 284.4937) -> (69.95, 328)
  line L2 (69.95, 328) -> (-71, 328)
  line L3 (-71, 328) -> (-71, 0)
  line L4 (-71, 0) -> (3, 0)
  line L5 (3, 0) -> (3, 279.5)
  arc A1 (11, 287.5) -> (3, 279.5) centre (11, 279.5) ccw
  line L6 (61.2, 333) -> (-71, 333)
  line L7 (-71, 333) -> (-71, 328)
  line L8 (-71, 328) -> (61.2, 328)
  line L9 (61.2, 328) -> (61.2, 333)
  point P0 (61.2, 333)
  constraint horizontal L6
  constraint vertical L7
  constraint horizontal L8
  constraint vertical L9
  constraint coincident L2.end L3.start
  constraint coincident P0 L6.start
extrude "Extrude238" add sketch "Sketch99" along normal blind 5 separate body makes body 12
sketch "Sketch100" plane through (-245, 0, 0) normal (1, 0, 0) x (0, 0, -1)
  line L0 (-56.2, 277.5) -> (-56.2, 317.5)
  line L1 (-56.2, 317.5) -> (-76.2, 317.5)
  line L2 (-76.2, 317.5) -> (-76.2, 213.5)
  line L3 (-76.2, 213.5) -> (-69.7, 213.5)
  line L4 (-69.7, 213.5) -> (-69.7, 277.5)
  line L5 (-69.7, 277.5) -> (-56.2, 277.5)
  line L6 (-56.2, 317.5) -> (-69.7, 317.5)
  line L7 (-69.7, 317.5) -> (-69.7, 277.5)
  line L8 (-69.7, 277.5) -> (-56.2, 277.5)
  line L9 (-56.2, 277.5) -> (-56.2, 317.5)
  constraint horizontal L6
  constraint vertical L7
  constraint horizontal L8
  constraint vertical L9
  constraint coincident L4.end L5.start
  constraint coincident L0.end L1.start
extrude "Extrude239" cut sketch "Sketch100" against normal blind 5 contours L0 L1 L5 L6 L7 L8 L9 bodies 8
extrude "Extrude240" cut 1 faces at (-289.7333, 277.5, 44.5333) along direction (0, 1, 0) blind 5 on bodies 8 bodies 8
extrude "Extrude241" add 1 faces at (-64, 247.6667, 56.2) along direction (0, 0, -1) blind 5 on bodies 8 bodies 8
extrude "Extrude242" cut 1 faces at (-235.8832, 318.8352, 68.7) along direction (0, 0, -1) blind 5 on bodies 8 bodies 8
extrude "Extrude243" cut 1 faces at (-237.5, 329.6667, 68.7) along direction (0, 0, -1) blind 5 on bodies 11 bodies 11
extrude "Extrude244" cut 1 faces at (-80.5, 329.6667, 68.7) along direction (0, 0, -1) blind 5 on bodies 11 bodies 11
extrude "Extrude245" cut 1 faces at (-79.1168, 318.8352, 68.7) along direction (0, 0, -1) blind 5 on bodies 8 bodies 8
extrude "Extrude246" cut 1 faces at (-235.8333, 197.1667, 68.7) along direction (0, 0, -1) blind 5 on bodies 8 bodies 8
extrude "Extrude247" cut 1 faces at (-79.1667, 197.1667, 68.7) along direction (0, 0, -1) blind 5 on bodies 8 bodies 8
extrude "Extrude248" add 1 faces at (-290.2667, 233.5, 71.7) along direction (0, 0, 1) blind 5 on bodies 8 bodies 8
extrude "Extrude249" cut 1 faces at (-151.6667, 210.8333, 68.7) along direction (0, 0, -1) blind 15 on bodies 8 bodies 8
extrude "Extrude250" cut sketch "Sketch84" against normal blind 3 bodies 7 8
extrude "Extrude251" cut 1 faces at (-289.7333, 282.5, 42.8667) along direction (0, 1, 0) blind 15 on bodies 8 bodies 8 12
extrude "Extrude252" cut 1 faces at (-307.6, 237.1458, 29.4667) along direction (-1, 0, 0) blind 10 on bodies 8 bodies 8
extrude "Extrude253" cut 1 faces at (-275.6292, 258.9292, 7.7) along direction (0, 0, -1) blind 5 on bodies 8 bodies 8 12
sketch "Sketch101" plane through (0, 0, 69.7) normal (0, 0, -1) x (-1, 0, 0)
  line L0 (245, 317.5) -> (245, 213.5)
  line L1 (245, 213.5) -> (311.8915, 213.5)
  line L2 (311.8915, 213.5) -> (311.8915, 279.5)
  arc A0 (311.8915, 279.5) -> (306.6, 284.7915) centre (306.6, 279.5) ccw
  line L3 (306.6, 284.7915) -> (259, 284.7915)
  line L4 (259, 284.7915) -> (259, 297.5)
  line L5 (259, 297.5) -> (250, 297.5)
  line L6 (250, 297.5) -> (250, 317.5)
  line L7 (250, 317.5) -> (245, 317.5)
  line L8 (259, 284.7915) -> (259, 213.5)
  constraint coincident L3.end L4.start
  constraint coincident L1 L8.end
  constraint perpendicular L1 L8
extrude "Extrude254" cut sketch "Sketch101" against normal blind 10 contours L1 L2 A0 L3 L8 bodies 8 12
sketch "Sketch102" plane through (0, 210.5, 0) normal (0, 1, 0) x (-1, 0, 0)
  arc A0 (314.6, 63.7) -> (306.6, 71.7) centre (306.6, 63.7) ccw
  line L0 (306.6, 71.7) -> (257.6, 71.7)
  line L1 (257.6, 71.7) -> (245, 71.7)
  line L2 (245, 71.7) -> (245, 76.2)
  line L3 (245, 76.2) -> (240.5, 76.2)
  line L4 (240.5, 76.2) -> (240.5, 63.7)
  line L5 (240.5, 63.7) -> (231.5, 63.7)
  line L6 (231.5, 63.7) -> (231.5, 76.2)
  line L7 (231.5, 76.2) -> (175, 76.2)
  line L8 (175, 76.2) -> (175, 53.7)
  line L9 (175, 53.7) -> (140, 53.7)
  line L10 (140, 53.7) -> (140, 76.2)
  line L11 (140, 76.2) -> (83.5, 76.2)
  line L12 (83.5, 76.2) -> (83.5, 63.7)
  line L13 (83.5, 63.7) -> (74.5, 63.7)
  line L14 (74.5, 63.7) -> (74.5, 76.2)
  line L15 (74.5, 76.2) -> (70, 76.2)
  line L16 (70, 76.2) -> (70, 51.2)
  line L17 (70, 51.2) -> (254, 51.2)
  line L18 (254, 51.2) -> (254, 20)
  line L19 (254, 20) -> (245, 20)
  line L20 (245, 20) -> (245, 15.5)
  line L21 (245, 15.5) -> (247, 15.5)
  line L22 (247, 15.5) -> (247, 10)
  line L23 (247, 10) -> (254, 10)
  line L24 (254, 10) -> (254, 2.7)
  line L25 (254, 2.7) -> (259, 2.7)
  line L26 (259, 2.7) -> (259, 3)
  line L27 (259, 3) -> (306.6, 3)
  arc A1 (306.6, 3) -> (307.6, 3.0627) centre (306.6, 11) ccw
  arc A2 (307.6, 3.0627) -> (314.6, 11) centre (306.6, 11) ccw
  line L28 (314.6, 11) -> (314.6, 63.7)
  line L29 (270, 55.7) -> (279, 55.7)
  line L30 (279, 55.7) -> (279, 36.1286)
  line L31 (279, 36.1286) -> (270, 45.1607)
  line L32 (270, 45.1607) -> (270, 55.7)
  line L33 (264, 2.7) -> (264, 71.7)
  point P0 (264, 2.7)
  constraint coincident P0 L33.start
  constraint coincident L0 L33.end
  constraint perpendicular L0 L33
extrude "Extrude255" cut sketch "Sketch102" against normal blind 5 contours A0 L0 L27 A1 A2 L28 L33 | L29 L30 L31 L32 bodies 7 8
extrude "Extrude256" add 1 faces at (-246.5, 198.8333, 76.2) along direction (0, 0, 1) blind 10 on bodies 8 bodies 8 12 7 11
extrude "Extrude257" add 1 faces at (-245, 329.6667, 76.2) along direction (0, 0, 1) blind 10 on bodies 8 bodies 8
extrude "Extrude258" cut 1 faces at (-251.3333, 241.5, 69.7) along direction (0, 0, 1) blind 10 on bodies 8 bodies 8
extrude "Extrude259" cut 1 faces at (-262.3333, 289.0277, 69.7) along direction (0, 0, 1) blind 2 on bodies 12 bodies 12
extrude "Extrude260" add 1 faces at (-260.6667, 328, 67.0333) along direction (0, 1, 0) blind 5 on bodies 12 bodies 12 8
sketch "Sketch103" plane through (0, 210.5, 0) normal (0, 1, 0) x (-1, 0, 0)
  line L0 (264, 2.7) -> (264, 71.7)
  line L1 (264, 71.7) -> (257.6, 71.7)
  line L2 (257.6, 71.7) -> (245, 71.7)
  line L3 (245, 71.7) -> (245, 86.2)
  line L4 (245, 86.2) -> (240.5, 86.2)
  line L5 (240.5, 86.2) -> (240.5, 63.7)
  line L6 (240.5, 63.7) -> (231.5, 63.7)
  line L7 (231.5, 63.7) -> (231.5, 76.2)
  line L8 (231.5, 76.2) -> (175, 76.2)
  line L9 (175, 76.2) -> (175, 53.7)
  line L10 (175, 53.7) -> (140, 53.7)
  line L11 (140, 53.7) -> (140, 76.2)
  line L12 (140, 76.2) -> (83.5, 76.2)
  line L13 (83.5, 76.2) -> (83.5, 63.7)
  line L14 (83.5, 63.7) -> (74.5, 63.7)
  line L15 (74.5, 63.7) -> (74.5, 76.2)
  line L16 (74.5, 76.2) -> (70, 76.2)
  line L17 (70, 76.2) -> (70, 51.2)
  line L18 (70, 51.2) -> (254, 51.2)
  line L19 (254, 51.2) -> (254, 20)
  line L20 (254, 20) -> (245, 20)
  line L21 (245, 20) -> (245, 15.5)
  line L22 (245, 15.5) -> (247, 15.5)
  line L23 (247, 15.5) -> (247, 10)
  line L24 (247, 10) -> (254, 10)
  line L25 (254, 10) -> (254, 2.7)
  line L26 (254, 2.7) -> (264, 2.7)
  line L27 (254, 2.7) -> (264, 2.7)
  line L28 (264, 2.7) -> (264, 71.7)
  line L29 (264, 71.7) -> (254, 71.7)
  line L30 (254, 71.7) -> (254, 2.7)
  constraint horizontal L27
  constraint vertical L28
  constraint horizontal L29
  constraint vertical L30
  constraint coincident L0.end L1.start
  constraint coincident L25.end L26.start
extrude "Extrude261" cut sketch "Sketch103" against normal blind 5 contours L0 L1 L2 L19 L25 L26 L27 L28 L29 L30 bodies 12
extrude "Extrude262" cut 1 faces at (-251.6667, 210.5, 15.1667) along direction (0, -1, 0) blind 5 on bodies 12 bodies 12
extrude "Extrude263" cut 1 faces at (-237.6667, 213.5, 15.1667) along direction (0, -1, 0) blind 8 on bodies 12 bodies 12
extrude "Extrude264" cut 1 faces at (-248, 213.5, 75.8667) along direction (0, -1, 0) blind 3 on bodies 12 bodies 12
sketch "Sketch104" plane through (0, 297.5, 0) normal (0, -1, 0) x (1, 0, 0)
  line L0 (-264, 69.95) -> (-264, 7.7)
  line L1 (-264, 7.7) -> (-259, 7.7)
  line L2 (-259, 7.7) -> (-259, 2.7)
  line L3 (-259, 2.7) -> (-254, 2.7)
  line L4 (-254, 2.7) -> (-254, 51.2)
  line L5 (-254, 51.2) -> (-250, 51.2)
  line L6 (-250, 51.2) -> (-250, 79.7)
  line L7 (-250, 79.7) -> (-254, 79.7)
  line L8 (-254, 79.7) -> (-254, 76.2)
  line L9 (-254, 76.2) -> (-259, 69.95)
  line L10 (-259, 69.95) -> (-264, 69.95)
  line L11 (-264, 69.95) -> (-254, 69.95)
  line L12 (-254, 69.95) -> (-254, 79.7)
  line L13 (-254, 79.7) -> (-264, 79.7)
  line L14 (-264, 79.7) -> (-264, 69.95)
  constraint horizontal L11
  constraint vertical L12
  constraint horizontal L13
  constraint vertical L14
  constraint coincident L7.end L8.start
  constraint coincident L0.start L10.end
extrude "Extrude265" add sketch "Sketch104" against normal blind 35.5 separate body contours L8 L9 L10 L11 L12 L13 L14 makes body 13
extrude "Extrude266" cut 1 faces at (-290.2667, 213.5, 75.0333) along direction (0, -1, 0) blind 5 on bodies 12 bodies 12
extrude "Extrude267" add 1 faces at (-270.6667, 205.5, 19.7095) along direction (0, 1, 0) blind 5 on bodies 12 bodies 12
sketch "Sketch105" plane through (0, 210.5, 0) normal (0, 1, 0) x (-1, 0, 0)
  line L0 (254, 51.2) -> (254, 20)
  line L1 (254, 20) -> (236, 20)
  line L2 (236, 20) -> (236, 10)
  line L3 (236, 10) -> (241, 10)
  line L4 (241, 10) -> (241, 15.5)
  line L5 (241, 15.5) -> (247, 15.5)
  line L6 (247, 15.5) -> (247, 10)
  line L7 (247, 10) -> (254, 10)
  line L8 (254, 10) -> (254, 2.7)
  line L9 (254, 2.7) -> (264, 2.7)
  line L10 (264, 2.7) -> (264, 3)
  line L11 (264, 3) -> (279, 3)
  line L12 (279, 3) -> (279, 36.1286)
  line L13 (279, 36.1286) -> (270, 45.1607)
  line L14 (270, 45.1607) -> (270, 56.2)
  line L15 (270, 56.2) -> (254, 76.2)
  line L16 (254, 76.2) -> (254, 79.7)
  line L17 (254, 79.7) -> (245, 79.7)
  line L18 (245, 79.7) -> (245, 86.2)
  line L19 (245, 86.2) -> (240.5, 86.2)
  line L20 (240.5, 86.2) -> (240.5, 63.7)
  line L21 (240.5, 63.7) -> (231.5, 63.7)
  line L22 (231.5, 63.7) -> (231.5, 76.2)
  line L23 (231.5, 76.2) -> (175, 76.2)
  line L24 (175, 76.2) -> (175, 53.7)
  line L25 (175, 53.7) -> (140, 53.7)
  line L26 (140, 53.7) -> (140, 76.2)
  line L27 (140, 76.2) -> (83.5, 76.2)
  line L28 (83.5, 76.2) -> (83.5, 63.7)
  line L29 (83.5, 63.7) -> (74.5, 63.7)
  line L30 (74.5, 63.7) -> (74.5, 76.2)
  line L31 (74.5, 76.2) -> (70, 76.2)
  line L32 (70, 76.2) -> (70, 51.2)
  line L33 (70, 51.2) -> (254, 51.2)
  line L34 (279, 36.1286) -> (254, 36.1286)
  line L35 (254, 36.1286) -> (254, 79.7)
  line L36 (254, 79.7) -> (279, 79.7)
  line L37 (279, 79.7) -> (279, 36.1286)
  constraint horizontal L34
  constraint vertical L35
  constraint horizontal L36
  constraint vertical L37
  constraint coincident L16.end L17.start
  constraint coincident L12.end L13.start
extrude "Extrude268" add sketch "Sketch105" against normal blind 10 separate body contours L13 L14 L15 L16 L35 L36 L37 makes body 14
extrude "Extrude269" add 1 faces at (-254, 321.1667, 80.7) along direction (-1, 0, 0) blind 60 on bodies 12 bodies 12 13 14
extrude "Extrude270" cut 1 faces at (-256, 297.5, 69.0333) along direction (0, 1, 0) blind 20 on bodies 12 bodies 12
extrude "Extrude271" cut 1 faces at (-262.3333, 297.0251, 7.7) along direction (0, 0, -1) blind 5 on bodies 12 bodies 12
sketch "Sketch106" plane through (0, 210.5, 0) normal (0, 1, 0) x (-1, 0, 0)
  line L0 (314, 79.7) -> (245, 79.7)
  line L1 (245, 79.7) -> (245, 86.2)
  line L2 (245, 86.2) -> (240.5, 86.2)
  line L3 (240.5, 86.2) -> (240.5, 63.7)
  line L4 (240.5, 63.7) -> (231.5, 63.7)
  line L5 (231.5, 63.7) -> (231.5, 76.2)
  line L6 (231.5, 76.2) -> (175, 76.2)
  line L7 (175, 76.2) -> (175, 53.7)
  line L8 (175, 53.7) -> (140, 53.7)
  line L9 (140, 53.7) -> (140, 76.2)
  line L10 (140, 76.2) -> (83.5, 76.2)
  line L11 (83.5, 76.2) -> (83.5, 63.7)
  line L12 (83.5, 63.7) -> (74.5, 63.7)
  line L13 (74.5, 63.7) -> (74.5, 76.2)
  line L14 (74.5, 76.2) -> (70, 76.2)
  line L15 (70, 76.2) -> (70, 51.2)
  line L16 (70, 51.2) -> (254, 51.2)
  line L17 (254, 51.2) -> (254, 20)
  line L18 (254, 20) -> (236, 20)
  line L19 (236, 20) -> (236, 10)
  line L20 (236, 10) -> (241, 10)
  line L21 (241, 10) -> (241, 15.5)
  line L22 (241, 15.5) -> (247, 15.5)
  line L23 (247, 15.5) -> (247, 10)
  line L24 (247, 10) -> (254, 10)
  line L25 (254, 10) -> (254, 2.7)
  line L26 (254, 2.7) -> (264, 2.7)
  line L27 (264, 2.7) -> (264, 3)
  line L28 (264, 3) -> (279, 3)
  line L29 (279, 3) -> (279, 76.2)
  line L30 (279, 76.2) -> (314, 76.2)
  line L31 (314, 76.2) -> (314, 79.7)
  line L32 (236, 20) -> (279, 20)
  line L33 (279, 20) -> (279, 15.5)
  line L34 (279, 15.5) -> (236, 15.5)
  line L35 (236, 15.5) -> (236, 20)
  line L36 (279, 3) -> (254, 3)
  line L37 (254, 3) -> (254, 20)
  line L38 (254, 20) -> (279, 20)
  line L39 (279, 20) -> (279, 3)
  constraint horizontal L32
  constraint vertical L33
  constraint horizontal L34
  constraint vertical L35
  constraint coincident L29 L33.end
  constraint coincident L18.end L19.start
  constraint horizontal L36
  constraint vertical L37
  constraint horizontal L38
  constraint vertical L39
  constraint coincident L17.end L18.start
  constraint coincident L28.end L29.start
extrude "Extrude272" add sketch "Sketch106" along normal blind 107 separate body contours L25 L28 L29 L34 L36 L37 L39 makes body 15
sketch "Sketch107" plane through (0, 210.5, 0) normal (0, 1, 0) x (-1, 0, 0)
  line L0 (314, 79.7) -> (245, 79.7)
  line L1 (245, 79.7) -> (245, 86.2)
  line L2 (245, 86.2) -> (240.5, 86.2)
  line L3 (240.5, 86.2) -> (240.5, 63.7)
  line L4 (240.5, 63.7) -> (231.5, 63.7)
  line L5 (231.5, 63.7) -> (231.5, 76.2)
  line L6 (231.5, 76.2) -> (175, 76.2)
  line L7 (175, 76.2) -> (175, 53.7)
  line L8 (175, 53.7) -> (140, 53.7)
  line L9 (140, 53.7) -> (140, 76.2)
  line L10 (140, 76.2) -> (83.5, 76.2)
  line L11 (83.5, 76.2) -> (83.5, 63.7)
  line L12 (83.5, 63.7) -> (74.5, 63.7)
  line L13 (74.5, 63.7) -> (74.5, 76.2)
  line L14 (74.5, 76.2) -> (70, 76.2)
  line L15 (70, 76.2) -> (70, 51.2)
  line L16 (70, 51.2) -> (254, 51.2)
  line L17 (254, 51.2) -> (254, 20)
  line L18 (254, 20) -> (236, 20)
  line L19 (236, 20) -> (236, 10)
  line L20 (236, 10) -> (241, 10)
  line L21 (241, 10) -> (241, 15.5)
  line L22 (241, 15.5) -> (247, 15.5)
  line L23 (247, 15.5) -> (247, 10)
  line L24 (247, 10) -> (254, 10)
  line L25 (254, 10) -> (254, 2.7)
  line L26 (254, 2.7) -> (264, 2.7)
  line L27 (264, 2.7) -> (264, 3)
  line L28 (264, 3) -> (279, 3)
  line L29 (279, 3) -> (279, 76.2)
  line L30 (279, 76.2) -> (314, 76.2)
  line L31 (314, 76.2) -> (314, 79.7)
  line L32 (236, 20) -> (279, 20)
  line L33 (279, 20) -> (279, 15.5)
  line L34 (279, 15.5) -> (236, 15.5)
  line L35 (236, 15.5) -> (236, 20)
  line L36 (254, 20) -> (279, 20)
  line L37 (279, 20) -> (279, 15.5)
  line L38 (279, 15.5) -> (254, 15.5)
  line L39 (254, 15.5) -> (254, 20)
  point P0 (279, 15.5)
  constraint horizontal L32
  constraint vertical L33
  constraint horizontal L34
  constraint vertical L35
  constraint coincident P0 L33.end
  constraint coincident L18.end L19.start
  constraint horizontal L36
  constraint vertical L37
  constraint horizontal L38
  constraint vertical L39
  constraint coincident L17.end L18.start
extrude "Extrude273" add sketch "Sketch107" along normal blind 107 contours L29 L32 L33 L34 L36 L37 L38 L39 bodies 15 12
extrude "Extrude274" add 1 faces at (-280.6667, 327.8333, 76.2) along direction (0, 0, -1) blind 73.2 on bodies 15 bodies 15
sketch "Sketch108" plane through (-279, 0, 0) normal (-1, 0, 0) x (0, 0, 1)
  line L0 (20, 317.5) -> (3, 317.5)
  line L1 (3, 317.5) -> (3, 0)
  line L2 (3, 0) -> (36.1286, 0)
  line L3 (36.1286, 0) -> (36.1286, 200.5)
  line L4 (36.1286, 200.5) -> (76.2, 200.5)
  line L5 (76.2, 200.5) -> (76.2, 210.5)
  line L6 (76.2, 210.5) -> (20, 210.5)
  line L7 (20, 210.5) -> (20, 317.5)
  line L8 (76.2, 210.5) -> (36.1286, 210.5)
  line L9 (36.1286, 210.5) -> (36.1286, 200.5)
  line L10 (36.1286, 200.5) -> (76.2, 200.5)
  line L11 (76.2, 200.5) -> (76.2, 210.5)
  constraint horizontal L8
  constraint vertical L9
  constraint horizontal L10
  constraint vertical L11
  constraint coincident L3.end L4.start
  constraint coincident L5.end L6.start
extrude "Extrude275" add sketch "Sketch108" along normal blind 35 separate body contours L4 L5 L6 L8 L9 L10 L11 makes body 16